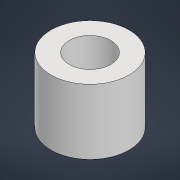
# Autodesk Inventor part: CU-305
Saved by Autodesk Inventor 2022.5 (Build 265521000, 521)
## iProperties
Created: 2022-03-25
Part Number: CU-305
Material: SUS304
Document SubType Name: Modeling
Designer: masayuki
Density: 7.93 g/cm^3
Appearance: 一般
Mass: 0.802193 g
Surface Area: 1.84977 cm^2
Volume: 0.101159 cm^3
Author: masayuki
Autodesk Inventor part; units mm, degrees
ref_plane "YZ Plane" through (0, 0, 0) normal (1, 0, 0) x (0, 1, 0)
ref_plane "XZ Plane" through (0, 0, 0) normal (0, 1, 0) x (-1, 0, 0)
ref_plane "XY Plane" through (0, 0, 0) normal (0, 0, 1) x (1, 0, 0)
sketch "スケッチ1" plane through (0, 0, 0) normal (0, 1, 0) x (-1, 0, 0)
  circle A0 centre (0, 0) radius 3
  dimension "d0" = 6
  constraints: 1 centre point, 1 coincident
  measures "d0" diameter of A0
extrude "押し出し1" add sketch "スケッチ1" along normal blind 5
sketch "スケッチ2" plane through (0, 5, 0) normal (0, 1, 0) x (1, 0, 0)
  circle A0 centre (0, 0) radius 1.6
  dimension "d3" = 3.2
  constraints: 1 centre point, 1 coincident
  measures "d3" diameter of A0
extrude "押し出し2" cut sketch "スケッチ2" against normal through all
